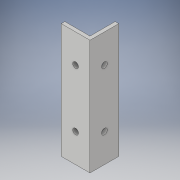
# Autodesk Inventor part: L Bracket 4in
Saved by Autodesk Inventor 2018 (Build 220112000, 112)
## iProperties
Created: 2018-01-19
Part Number: L Bracket 4in
Material: Generic
Document SubType Name: Modeling
Designer: S-2512711
Density: 1 g/cm^3
Appearance: Default
Author: S-2512711
Autodesk Inventor part; units mm, degrees
ref_plane "YZ Plane" through (0, 0, 0) normal (1, 0, 0) x (0, 1, 0)
ref_plane "XZ Plane" through (0, 0, 0) normal (0, 1, 0) x (-1, 0, 0)
ref_plane "XY Plane" through (0, 0, 0) normal (0, 0, 1) x (1, 0, 0)
sketch "Sketch1" plane through (0, 0, 0) normal (0, 1, 0) x (-1, 0, 0)
  line L0 (0, 0) -> (-25.4, 0)
  line L1 (-25.4, 0) -> (-25.4, -3.175)
  line L2 (-25.4, -3.175) -> (0, -3.175)
  line L3 (0, -3.175) -> (0, 0)
  line L4 (-25.4, 0) -> (-22.225, 0)
  line L5 (-22.225, 0) -> (-22.225, -25.4)
  line L6 (-22.225, -25.4) -> (-25.4, -25.4)
  line L7 (-25.4, -25.4) -> (-25.4, 0)
  dimension "d0" = 25.4
  dimension "d1" = 3.175
  dimension "d2" = 25.4
  dimension "d3" = 3.175
  constraints: 16 end point, 4 parallel, 2 horizontal, 2 perpendicular
  measures "d0" distance of L2.end L1.end
  measures "d1" distance of L5.end L6.end
  measures "d2" distance of L6.end L0.end
  measures "d3" distance of L2.end L0.start
extrude "Extrusion1" add sketch "Sketch1" along normal blind 101.6
sketch "Sketch2" plane through (25.4, 0, 0) normal (1, 0, 0) x (0, 0, -1)
  line L0 (0, 0) -> (0, 101.6) projected
  line L1 (0, 101.6) -> (12.7, 101.6)
  line L2 (25.4, 101.6) -> (3.175, 101.6) projected
  line L3 (12.7, 101.6) -> (12.7, 76.2)
  line L4 (0, 0) -> (12.7, 0)
  line L5 (0, 0) -> (25.4, 0) projected
  line L6 (12.7, 0) -> (12.7, 25.4)
  circle A0 centre (12.7, 76.2) radius 2.54
  circle A1 centre (12.7, 25.4) radius 2.54
  dimension "d6" = 12.7
  dimension "d7" = 25.4
  dimension "d8" = 25.4
  dimension "d9" = 5.08
  constraints: 8 end point, 2 centre point, 2 coincident, 2 perpendicular, 1 midpoint, 1 point on line
  measures "d6" distance of L0.end L1.end
  measures "d7" distance of L1.end L3.end
  measures "d8" distance of L4.end L6.end
  measures "d9" diameter of A0
extrude "Extrusion2" cut sketch "Sketch2" against normal blind 25.4
sketch "Sketch3" plane through (0, 0, 0) normal (0, 0, 1) x (1, 0, 0)
  line L0 (0, 0) -> (0, 101.6) projected
  line L1 (0, 0) -> (12.7, 0)
  line L2 (0, 0) -> (25.4, 0) projected
  line L3 (12.7, 0) -> (12.7, 25.4)
  line L4 (0, 101.6) -> (25.4, 101.6) projected
  line L5 (12.7, 101.6) -> (12.7, 76.2)
  circle A0 centre (12.7, 76.2) radius 2.54
  circle A1 centre (12.7, 25.4) radius 2.54
  dimension "d12" = 25.4
  dimension "d13" = 25.4
  dimension "d14" = 5.08
  constraints: 6 end point, 2 centre point, 2 coincident, 2 midpoint, 1 perpendicular, 1 vertical
  measures "d12" distance of L1.end L3.end
  measures "d13" distance of L5.start L5.end
  measures "d14" diameter of A0
extrude "Extrusion3" cut sketch "Sketch3" against normal blind 25.4
body "Solid1"
